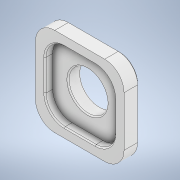
# Autodesk Inventor part: Capinsert_back
Saved by Autodesk Inventor 2021 (Build 250183000, 183)
## iProperties
Created: 2022-04-22
Part Number: Capinsert_back
Material: PPS-Kunststoff
Document SubType Name: Modeling
Designer: Timo
Density: 1.637 g/cm^3
Appearance: Glatt - Weiß
Mass: 1.91867 g
Surface Area: 13.5025 cm^2
Volume: 1.17207 cm^3
Author: Timo
Autodesk Inventor part; units mm, degrees
ref_plane "YZ Plane" through (0, 0, 0) normal (1, 0, 0) x (0, 1, 0)
ref_plane "XZ Plane" through (0, 0, 0) normal (0, 1, 0) x (-1, 0, 0)
ref_plane "XY Plane" through (0, 0, 0) normal (0, 0, 1) x (1, 0, 0)
sketch "Skizze1" plane through (0, 0, 0) normal (0, 0, 1) x (1, 0, 0)
  line L0 (-11.45, -11.45) -> (11.45, -11.45)
  line L1 (11.45, -11.45) -> (11.45, 11.45)
  line L2 (11.45, 11.45) -> (-11.45, 11.45)
  line L3 (-11.45, 11.45) -> (-11.45, -11.45)
  line L4 (-11.45, -11.45) -> (11.45, 11.45) construction
  line L5 (11.45, -11.45) -> (-11.45, 11.45) construction
  point P0 (0, 0)
  dimension "d0" = 22.9
  constraints: 12 end point, 2 midpoint, 2 parallel, 2 perpendicular, 1 horizontal
  measures "d0" distance of L2.end L1.end
extrude "Extrusion1" add sketch "Skizze1" along normal blind 3.8
fillet "Rundung1" radius 5 4 edges at (11.45, 11.45, 1.9) (11.45, -11.45, 1.9) (-11.45, -11.45, 1.9) (-11.45, 11.45, 1.9)
sketch "Skizze2" plane through (0, 0, 3.8) normal (0, 0, 1) x (1, 0, 0)
  line L0 (-8.99, -8.99) -> (8.99, -8.99)
  line L1 (8.99, -8.99) -> (8.99, 8.99)
  line L2 (8.99, 8.99) -> (-8.99, 8.99)
  line L3 (-8.99, 8.99) -> (-8.99, -8.99)
  line L4 (-8.99, -8.99) -> (8.99, 8.99) construction
  line L5 (8.99, -8.99) -> (-8.99, 8.99) construction
  point P0 (0, 0)
  dimension "d5" = 17.98
  constraints: 12 end point, 2 midpoint, 2 parallel, 2 perpendicular, 1 horizontal
  measures "d5" distance of L2.end L1.end
extrude "Extrusion2" cut sketch "Skizze2" against normal blind 2
fillet "Rundung2" radius 5 4 edges at (-8.99, 8.99, 2.8) (8.99, 8.99, 2.8) (-8.99, -8.99, 2.8) (8.99, -8.99, 2.8)
sketch "Skizze3" plane through (0, 0, 1.8) normal (0, 0, 1) x (1, 0, 0)
  circle A0 centre (0, 0) radius 5.025
  line L0 (-3.55, -3.5564) -> (3.55, -3.5564) construction
  line L1 (3.55, -3.5564) -> (3.55, 3.5564)
  line L2 (3.55, 3.5564) -> (-3.55, 3.5564) construction
  line L3 (-3.55, 3.5564) -> (-3.55, -3.5564)
  line L4 (-3.55, -3.5564) -> (3.55, 3.5564) construction
  line L5 (3.55, -3.5564) -> (-3.55, 3.5564) construction
  point P0 (-3.55, 3.5564)
  point P1 (-3.55, -3.5564)
  point P2 (3.55, -3.5564)
  dimension "d10" = 10.05
  dimension "d11" = 7.1
  constraints: 12 end point, 2 midpoint, 2 parallel, 1 coincident, 1 horizontal, 1 perpendicular, 3 other
  measures "d11" distance of L2.end L1.end
extrude "Extrusion3" cut sketch "Skizze3" against normal through all
sketch "Skizze4" plane through (0, 0, 0) normal (0, 0, -1) x (-1, 0, 0)
  circle A0 centre (0, 0) radius 6.45
  circle A1 centre (0, 0) radius 5.025 projected
  dimension "d14" = 12.9
  constraints: 1 centre point, 1 coincident
  measures "d14" diameter of A0
extrude "Extrusion4" add sketch "Skizze4" along normal blind 1.5
chamfer "Fase1" distance 0.3 angle 45 8 edges at (0, 8.99, 3.8) (7.5255, 7.5255, 3.8) (8.99, 0, 3.8) (7.5255, -7.5255, 3.8) (0, -8.99, 3.8) (-7.5255, -7.5255, 3.8) (-8.99, 0, 3.8) (-7.5255, 7.5255, 3.8)
chamfer "Fase2" distance 0.3 angle 45 8 edges at (11.45, 0, 0) (9.9855, 9.9855, 0) (0, 11.45, 0) (-9.9855, 9.9855, 0) (-11.45, 0, 0) (-9.9855, -9.9855, 0) (0, -11.45, 0) (9.9855, -9.9855, 0)
fillet "Rundung3" radius 0.3 1 edges at (-3.55, 3.5564, 1.8)
fillet "Rundung4" radius 0.3 1 edges at (5.025, 0, -1.5)
